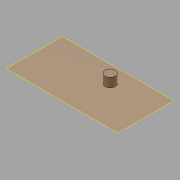
# Autodesk Inventor part: frame1b
Saved by Autodesk Inventor 2015 (Build 190159000, 159)
## iProperties
Created: 2017-01-17
Part Number: frame1b
Material: Generic
Document SubType Name: Modeling
Designer: Paulo Loma
Density: 1 g/cm^3
Appearance: Default
Author: Paulo Loma
Autodesk Inventor part; units mm, degrees
ref_plane "YZ Plane" through (0, 0, 0) normal (1, 0, 0) x (0, 1, 0)
ref_plane "XZ Plane" through (0, 0, 0) normal (0, 1, 0) x (-1, 0, 0)
ref_plane "XY Plane" through (0, 0, 0) normal (0, 0, 1) x (1, 0, 0)
ref_plane "Work Plane1" through (0, 0, 18) normal (0, 0, 1) x (1, 0, 0)
sketch "Sketch1" plane through (0, 0, 18) normal (0, 0, 1) x (1, 0, 0)
  circle A0 centre (0.9362, 6.0941) radius 2.5 projected
  circle A1 centre (0.9362, 6.0941) radius 1.25
  point P0 (0, 0)
  constraints: 1 centre point, 2 other
ref_plane "Work Plane2" through (-2.3703, 2.7876, 13.6) normal (0, 0, 1) x (0.9118791, -0.410459, 0)
ref_plane "Work Plane3" through (-2.3703, 2.7876, 13.6) normal (0, 0, 1) x (0.9118791, -0.410459, 0)
extrude "Extrusion2" add sketch "Sketch1" against normal up to surface (4.4 mm away)
sketch "Sketch2" plane through (0, 0, 18) normal (0, 0, 1) x (1, 0, 0)
  circle A0 centre (-11.0618, 6.3096) radius 2.15 projected
  point P0 (0, 0)
ref_plane "Work Plane4" through (-14.169, 3.2822, 13.9) normal (0, 0, 1) x (0.9992994, -0.0374251, 0)
extrude "Extrusion3" add sketch "Sketch2" against normal up to surface (4.1 mm away)
sketch "Sketch3" plane through (-11.0618, 6.3096, 13.9) normal (0, 0, -1) x (-1, 0, 0)
  circle A0 centre (0, 0) radius 1 projected
  point P0 (-11.0618, -6.3096)
extrude "Extrusion4" add sketch "Sketch3" along normal blind 10
sketch "Sketch4" plane through (0, 0, 18) normal (0, 0, 1) x (1, 0, 0)
  circle A0 centre (-20.9608, 0.4563) radius 2.15 projected
  point P0 (0, 0)
ref_plane "Work Plane5" through (-25.1421, -3.7287, 11.9) normal (0, 0, 1) x (0.7300141, 0.683432, 0)
extrude "Extrusion5" add sketch "Sketch4" against normal up to surface (6.1 mm away)
sketch "Sketch5" plane through (-20.9608, 0.4563, 11.9) normal (0, 0, -1) x (-1, 0, 0)
  circle A0 centre (0, 0) radius 1 projected
  point P0 (-20.9608, -0.4563)
extrude "Extrusion6" add sketch "Sketch5" along normal up to surface (8 mm away)
sketch "Sketch6" plane through (0, 0, 18) normal (0, 0, 1) x (1, 0, 0)
  line L0 (-18.7174, -15.8242) -> (-6.2675, -15.8242)
  arc A0 (-6.2675, -15.8242) -> (-4.8841, -15.2686) centre (-6.2675, -13.8242) ccw
  arc A1 (-4.8841, -15.2686) -> (-1.4924, -7.3242) centre (-12.4924, -7.3242) ccw
  line L1 (-1.4924, -7.3242) -> (4.745, -7.3242)
  arc A2 (7.8284, -0.102) -> (4.745, -7.3242) centre (14.745, -7.3242) ccw
  arc A3 (8.52, 0.1758) -> (7.8284, -0.102) centre (8.52, -0.8242) ccw
  line L2 (8.52, 0.1758) -> (20.9699, 0.1758)
  arc A4 (21.6616, -0.102) -> (20.9699, 0.1758) centre (20.9699, -0.8242) ccw
  arc A5 (24.2465, -4.2063) -> (21.6616, -0.102) centre (14.745, -7.3242) ccw
  line L3 (24.2465, -4.2063) -> (25.2939, -4.2063)
  line L4 (25.2939, -4.2063) -> (25.2939, 8.6758)
  line L5 (0.9362, 9.5941) -> (25.2939, 9.5941)
  line L6 (25.2939, 9.5941) -> (25.2939, 8.6758)
  line L7 (0.9362, 9.5941) -> (-33.0638, 9.5941)
  line L8 (-33.0638, 9.5941) -> (-33.0638, -7.3242)
  line L9 (-18.7174, -15.8242) -> (-24.5638, -15.8242)
  arc A6 (-33.0638, -7.3242) -> (-24.5638, -15.8242) centre (-24.5638, -7.3242) ccw projected
  point P0 (0, 0)
  constraints: 20 end point, 13 point on circle, 6 centre point, 1 horizontal, 1 vertical
extrude "Extrusion7" add sketch "Sketch6" against normal blind 1
sketch "Sketch7" plane through (0, 0, 17) normal (0, 0, -1) x (-1, 0, 0)
  arc A0 (4.8841, -15.2686) -> (6.2675, -15.8242) centre (6.2675, -13.8242) ccw
  arc A1 (1.4924, -7.3242) -> (4.8841, -15.2686) centre (12.4924, -7.3242) ccw
  line L0 (1.4924, -7.3242) -> (-4.745, -7.3242)
  arc A2 (-4.745, -7.3242) -> (-4.7951, -6.3242) centre (-14.745, -7.3242) ccw
  line L1 (-24.2465, -4.2063) -> (-25.2939, -4.2063)
  line L2 (-25.2939, -4.2063) -> (-25.2939, 9.5941)
  arc A3 (5.5758, -14.5464) -> (6.2675, -14.8242) centre (6.2675, -13.8242) ccw
  arc A4 (2.5425, -6.3242) -> (5.5758, -14.5464) centre (12.4924, -7.3242) ccw
  line L3 (2.5425, -6.3242) -> (-3.7905, -6.3242)
  line L4 (-13.2939, 9.5941) -> (-12.2465, 9.5941)
  line L5 (-24.2465, -4.2063) -> (-24.2465, 3.5941)
  line L6 (-24.2465, 4.5941) -> (-24.2465, 8.5941)
  line L7 (-3.7905, -6.3242) -> (-4.7951, -6.3242)
  line L8 (-24.2465, 3.5941) -> (-24.2465, 8.5941)
  arc A5 (24.5638, -14.8242) -> (32.0638, -7.3242) centre (24.5638, -7.3242) ccw projected
  arc A6 (24.5638, -15.8242) -> (33.0638, -7.3242) centre (24.5638, -7.3242) ccw projected
  line L9 (17.9156, -14.8242) -> (12.9156, -14.8242)
  line L10 (12.9156, -13.8242) -> (17.9156, -13.8242)
  line L11 (12.9156, -14.8242) -> (12.9156, -15.8242)
  line L12 (17.9156, -14.8242) -> (17.9156, -15.8242)
  line L13 (17.9156, -13.8242) -> (18.9156, -13.8242)
  line L14 (18.9156, -13.8242) -> (18.9156, -14.8242)
  line L15 (12.9156, -13.8242) -> (11.9156, -13.8242)
  line L16 (11.9156, -13.8242) -> (11.9156, -14.8242)
  line L17 (24.5638, -15.8242) -> (17.9156, -15.8242)
  line L18 (12.9156, -15.8242) -> (6.2675, -15.8242)
  line L19 (11.9156, -14.8242) -> (6.2675, -14.8242)
  line L20 (24.5638, -14.8242) -> (18.9156, -14.8242)
  line L21 (17.9156, -14.8242) -> (12.9156, -14.8242)
  line L22 (32.0638, -1.365) -> (32.0638, 3.635)
  line L23 (33.0638, 3.635) -> (32.0638, 3.635)
  line L24 (32.0638, 3.635) -> (32.0638, -1.365)
  line L25 (32.0638, -1.365) -> (33.0638, -1.365)
  line L26 (32.0638, -2.365) -> (31.0638, -2.365)
  line L27 (31.0638, -2.365) -> (31.0638, 4.635)
  line L28 (31.0638, 4.635) -> (32.0638, 4.635)
  line L29 (32.0638, -2.365) -> (32.0638, -7.3242)
  line L30 (32.0638, 8.5941) -> (32.0638, 4.635)
  line L31 (32.0638, 3.635) -> (32.0638, -1.365)
  line L32 (33.0638, 9.5941) -> (33.0638, 3.635)
  line L33 (33.0638, -1.365) -> (33.0638, -7.3242)
  line L34 (33.0638, 9.5941) -> (33.0638, 3.635)
  line L35 (33.0638, -1.365) -> (33.0638, -7.3242)
  line L36 (32.0638, 8.5941) -> (28.0638, 8.5941)
  line L37 (28.0638, 8.5941) -> (28.0638, 9.5941)
  line L38 (-12.2465, 8.5941) -> (-12.2465, 9.5941)
  line L39 (-20.7465, 9.5941) -> (-20.7465, 8.5941)
  line L40 (-20.7465, 8.5941) -> (-15.7465, 8.5941)
  line L41 (-15.7465, 8.5941) -> (-15.7465, 9.5941)
  line L42 (-14.7465, 7.5941) -> (-21.7465, 7.5941)
  line L43 (-21.7465, 7.5941) -> (-21.7465, 8.5941)
  line L44 (-14.7465, 8.5941) -> (-14.7465, 7.5941)
  line L45 (-24.2465, 8.5941) -> (-21.7465, 8.5941)
  line L46 (-20.7465, 8.5941) -> (-15.7465, 8.5941)
  line L47 (-14.7465, 8.5941) -> (-12.2465, 8.5941)
  line L48 (-25.2939, 9.5941) -> (-20.7465, 9.5941)
  line L49 (-15.7465, 9.5941) -> (33.0638, 9.5941)
  line L50 (33.0638, 9.5941) -> (-15.7465, 9.5941)
  line L51 (-20.7465, 9.5941) -> (-25.2939, 9.5941)
  line L52 (-25.2939, 9.5941) -> (-20.7465, 9.5941)
  line L53 (-15.7465, 9.5941) -> (33.0638, 9.5941)
  point P0 (0, 0)
  point P1 (32.0638, 9.5941)
  point P2 (-24.2465, 9.5941)
  point P3 (15.4156, -14.8242)
  point P4 (15.4156, -14.3242)
  point P5 (33.0638, 1.135)
  point P6 (32.5638, 1.135)
  point P7 (-18.2465, 8.5941)
  constraints: 108 end point, 22 perpendicular, 14 point on circle, 8 centre point, 6 horizontal, 5 point on line, 4 parallel, 2 midpoint, 2 vertical
extrude "Extrusion9" add sketch "Sketch7" along normal blind 8.5
sketch "Sketch11" plane through (0, 0, 8.5) normal (0, 0, -1) x (-1, 0, 0)
  line L0 (17.9156, -13.8242) -> (12.9156, -13.8242)
  line L1 (12.9156, -13.8242) -> (17.9156, -13.8242)
  line L2 (12.9156, -14.8242) -> (17.9156, -14.8242)
  line L3 (17.9156, -13.8242) -> (12.9156, -13.8242)
  line L4 (12.9156, -13.8242) -> (12.9156, -14.8242)
  line L5 (12.9156, -14.8242) -> (17.9156, -14.8242)
  line L6 (17.9156, -14.8242) -> (17.9156, -13.8242)
  line L7 (17.9156, -13.8242) -> (12.9156, -14.8242) construction
  line L8 (12.9156, -13.8242) -> (17.9156, -14.8242) construction
  line L9 (31.0638, 3.635) -> (31.0638, -1.365)
  line L10 (31.0638, -1.365) -> (31.0638, 3.635)
  line L11 (32.0638, -1.365) -> (32.0638, 3.635)
  line L12 (32.0638, 3.635) -> (31.0638, 3.635)
  line L13 (31.0638, 3.635) -> (31.0638, -1.365)
  line L14 (31.0638, -1.365) -> (32.0638, -1.365)
  line L15 (32.0638, -1.365) -> (32.0638, 3.635)
  line L16 (32.0638, 3.635) -> (31.0638, -1.365) construction
  line L17 (31.0638, 3.635) -> (32.0638, -1.365) construction
  line L18 (-20.7465, 7.5941) -> (-15.7465, 7.5941)
  line L19 (-15.7465, 7.5941) -> (-20.7465, 7.5941)
  line L20 (-15.7465, 8.5941) -> (-20.7465, 8.5941)
  line L21 (-15.7465, 8.5941) -> (-20.7465, 8.5941)
  line L22 (-20.7465, 8.5941) -> (-20.7465, 7.5941)
  line L23 (-20.7465, 7.5941) -> (-15.7465, 7.5941)
  line L24 (-15.7465, 7.5941) -> (-15.7465, 8.5941)
  line L25 (-15.7465, 8.5941) -> (-20.7465, 7.5941) construction
  line L26 (-20.7465, 8.5941) -> (-15.7465, 7.5941) construction
  point P0 (0, 0)
  point P1 (15.4156, -14.3242)
  point P2 (31.5638, 1.135)
  point P3 (-18.2465, 8.0941)
  constraints: 54 end point, 6 midpoint
extrude "Extrusion12" add sketch "Sketch11" along normal blind 6
sketch "Sketch12" plane through (-17.9156, -14.8242, 8.5) normal (-1, 0, 0) x (0, 0, 1)
  line L0 (-6, 0) -> (-3, 0)
  line L1 (0, 0) -> (-6, 0) projected
  line L2 (-3, 0) -> (-3, -1)
  line L3 (-3, -1) -> (-6, 0)
  point P0 (-8.5, 14.8242)
  dimension "d53" = 3
  dimension "d54" = 1
  constraints: 6 end point, 1 midpoint, 1 vertical
  measures "d53" distance of L0.start L0.end
  measures "d54" distance of L0.end L2.end
extrude "Extrusion13" add sketch "Sketch12" against normal blind 5
sketch "Sketch13" plane through (-32.0638, 3.635, 8.5) normal (0, 1, 0) x (1, 0, 0)
  line L0 (0, 6) -> (0, 3)
  line L1 (0, 0) -> (0, 6) projected
  line L2 (0, 3) -> (-1, 3)
  line L3 (-1, 3) -> (0, 6)
  point P0 (32.0638, 8.5)
  dimension "d57" = 3
  dimension "d58" = 1
  constraints: 6 end point, 1 midpoint, 1 perpendicular
  measures "d57" distance of L0.start L0.end
  measures "d58" distance of L0.end L2.end
extrude "Extrusion14" add sketch "Sketch13" against normal blind 5
sketch "Sketch14" plane through (20.7465, 7.5941, 8.5) normal (1, 0, 0) x (0, 0, -1)
  line L0 (6, 1) -> (3, 1)
  line L1 (0, 1) -> (6, 1) projected
  line L2 (3, 1) -> (3, 2)
  line L3 (3, 2) -> (6, 1)
  point P0 (8.5, -7.5941)
  dimension "d61" = 3
  dimension "d62" = 1
  constraints: 6 end point, 1 midpoint, 1 perpendicular
  measures "d61" distance of L0.start L0.end
  measures "d62" distance of L0.end L2.end
extrude "Extrusion15" add sketch "Sketch14" against normal blind 5
body "Solid2"
